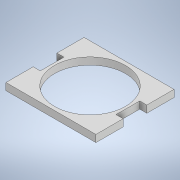
# Autodesk Inventor part: SoporteSensor
Saved by Autodesk Inventor 2020.2 (Build 242310000, 310)
## iProperties
Created: 2020-03-18
Part Number: SoporteSensor
Material: Generic
Document SubType Name: Modeling
Designer: ARQ SEVILLA R
Density: 1 g/cm^3
Appearance: Default
Author: ARQ SEVILLA R
Autodesk Inventor part; units mm, degrees
ref_plane "YZ Plane" through (0, 0, 0) normal (1, 0, 0) x (0, 1, 0)
ref_plane "XZ Plane" through (0, 0, 0) normal (0, 1, 0) x (-1, 0, 0)
ref_plane "XY Plane" through (0, 0, 0) normal (0, 0, 1) x (1, 0, 0)
sketch "Sketch1" plane through (0, 0, 0) normal (0, 1, 0) x (-1, 0, 0)
  line L0 (0, 0) -> (19, 0) construction
  line L1 (19, -5) -> (19, -15.5)
  line L2 (19, 0) -> (16, 0) construction
  line L3 (16, 0) -> (16, -5)
  line L4 (16, -5) -> (19, -5)
  circle A0 centre (0, 0) radius 14.5
  line L5 (19, -15.5) -> (0, -15.5)
  line L6 (0, 0) -> (0, 19.3776) construction
  line L7 (19, 5) -> (19, 15.5)
  line L8 (16, 0) -> (16, 5)
  line L9 (16, 5) -> (19, 5)
  line L10 (19, 15.5) -> (0, 15.5)
  line L11 (0, 0) -> (0, -19.3776) construction
  line L12 (-19, -5) -> (-19, -15.5)
  line L13 (-16, 0) -> (-16, -5)
  line L14 (-16, -5) -> (-19, -5)
  line L15 (-19, -15.5) -> (0, -15.5)
  line L16 (-16, 0) -> (-16, 5)
  line L17 (-16, 5) -> (-19, 5)
  line L18 (-19, 5) -> (-19, 15.5)
  line L19 (-19, 15.5) -> (0, 15.5)
  dimension "d1" = 19
  dimension "d2" = 15.5
  dimension "d5" = 5
  constraints: 40 end point, 12 symmetric about line, 3 perpendicular, 2 coincident, 2 horizontal, 1 centre point, 1 point on line, 1 vertical
  measures "d1" distance of L0.start L0.end
  measures "d2" distance of L0.end L1.end
  measures "d5" distance of L2.end L3.end
extrude "Extrusion1" add sketch "Sketch1" along normal blind 3 contours L1 L5 L15 L12 L14 L13 L16 L17 L18 L19 L10 L7 L9 L8 L3 L4 | A0
sketch "Sketch4" plane through (0, 3, 0) normal (0, 1, 0) x (1, 0, 0)
  circle A0 centre (0, 0) radius 15
  dimension "d14" = 30
  constraints: 1 centre point, 1 coincident
  measures "d14" diameter of A0
extrude "Extrusion4" cut sketch "Sketch4" against normal up to surface (3 mm away)
sketch "Sketch5" plane through (0, 0, 0) normal (0, -1, 0) x (1, 0, 0)
  line L0 (19, -15.5) -> (-19, -15.5) projected
  line L1 (-19, -15.5) -> (-19, -16.5)
  line L2 (-19, -16.5) -> (19, -16.5)
  line L3 (19, -16.5) -> (19, -15.5)
  line L4 (-19, 15.5) -> (19, 15.5) projected
  line L5 (19, 15.5) -> (19, 16.5)
  line L6 (19, 16.5) -> (-19, 16.5)
  line L7 (-19, 16.5) -> (-19, 15.5)
  point P0 (0, 0)
  dimension "d17" = 1
  dimension "d18" = 1
  constraints: 12 end point, 4 perpendicular, 2 vertical
  measures "d17" distance of L0.end L1.end
  measures "d18" distance of L4.end L5.end
extrude "Extrusion5" add sketch "Sketch5" against normal up to surface (3 mm away)
body "Solid1"
